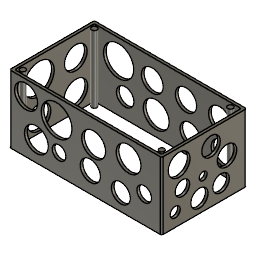
psu housing of anycibic kossel lienar plus_ (Autodesk Fusion 360 archive; units mm, degrees)
design "side_pannel"
part number: 2026-08-06-01-08-32-616
Autodesk Fusion 360 part; units mm, degrees
note: some values were not read from the file. Chosen so that the rebuilt part matches the saved one: which bodies a step acts on.
sketch "Sketch1" plane through (0, 0, 0) normal (0, 0, 1) x (1, 0, 0)
  line L0 (1, 0) -> (112, 0)
  line L1 (113, 0) -> (113, 63)
  line L2 (113, 63) -> (1, 63)
  line L3 (0, 63) -> (0, 1)
  line L4 (0, 0) -> (2, 0)
  line L5 (2, 3) -> (2, 60)
  line L6 (2, 63) -> (0, 63)
  line L7 (0, 62) -> (0, 0)
  line L8 (0, 0) -> (113, 0)
  line L9 (113, 0) -> (113, 2)
  line L10 (110, 2) -> (3, 2)
  line L11 (0, 2) -> (0, 0)
  line L12 (113, 63) -> (111, 63)
  line L13 (111, 60) -> (111, 3)
  line L14 (111, 0) -> (113, 0)
  line L15 (113, 1) -> (113, 62)
  line L16 (112, 63) -> (0, 63)
  line L17 (0, 63) -> (0, 61)
  line L18 (3, 61) -> (110, 61)
  line L19 (113, 61) -> (113, 63)
  arc A0 (112, 0) -> (113, 1) centre (112, 1) ccw
  arc A1 (113, 62) -> (112, 63) centre (112, 62) ccw
  arc A2 (1, 63) -> (0, 62) centre (1, 62) ccw
  arc A3 (0, 1) -> (1, 0) centre (1, 1) ccw
  arc A4 (3, 61) -> (2, 60) centre (3, 60) ccw
  arc A5 (2, 3) -> (3, 2) centre (3, 3) ccw
  arc A6 (110, 2) -> (111, 3) centre (110, 3) ccw
  arc A7 (111, 60) -> (110, 61) centre (110, 60) ccw
  dimension "d1" = 63
  dimension "d2" = 113
  dimension "d3" = 2
  dimension "d4" = 2
  dimension "d5" = 2
  dimension "d6" = 2
  dimension "d7" = 1
  dimension "d8" = 1
  constraint horizontal L0
  constraint vertical L1
  constraint horizontal L2
  constraint vertical L3
  constraint coincident L4.start L7.end
  constraint horizontal L4
  constraint vertical L5
  constraint horizontal L6
  constraint vertical L7
  constraint coincident L2 L6.start
  constraint horizontal L8
  constraint vertical L9
  constraint horizontal L10
  constraint vertical L11
  constraint coincident L1 L9.end
  constraint horizontal L12
  constraint vertical L13
  constraint horizontal L14
  constraint vertical L15
  constraint coincident L8 L14.start
  constraint horizontal L16
  constraint vertical L17
  constraint horizontal L18
  constraint vertical L19
  constraint coincident L7 L17.end
  constraint coincident L1.start L0
  constraint coincident L1.start L15
  constraint tangent L0 A0
  constraint tangent L15 A0
  constraint coincident L1.end L16
  constraint coincident L1.end L15
  constraint tangent L16 A1
  constraint tangent L15 A1
  constraint equal A0 A1
  constraint coincident L3.start L2
  constraint coincident L3.start L7
  constraint tangent L2 A2
  constraint tangent L7 A2
  constraint equal A0 A2
  constraint coincident L4.start L3
  constraint coincident L4.start L0
  constraint tangent L3 A3
  constraint tangent L0 A3
  constraint equal A0 A3
  constraint coincident L17.end L18
  constraint coincident L6.start L5
  constraint tangent L18 A4
  constraint tangent L5 A4
  constraint coincident L4.end L5
  constraint coincident L11.start L10
  constraint tangent L5 A5
  constraint tangent L10 A5
  constraint equal A4 A5
  constraint coincident L9.end L10
  constraint coincident L14.start L13
  constraint tangent L10 A6
  constraint tangent L13 A6
  constraint equal A4 A6
  constraint coincident L19.start L18
  constraint coincident L12.end L13
  constraint tangent L18 A7
  constraint tangent L13 A7
  constraint equal A4 A7
  measures "d1" distance of L4.start L3.start
  measures "d2" distance of L4.start L1.start
  measures "d3" distance of L3 L5
  measures "d4" distance of L0 L10
  measures "d5" distance of L13 L15
  measures "d6" distance of L2 L18
  measures "d7" radius of A0
  measures "d8" radius of A4
sketch "Sketch2" plane through (0, 0, 0) normal (0, 0, 1) x (1, 0, 0)
  circle A0 centre (108, 5) radius 2
  circle A1 centre (5, 5) radius 2
  circle A2 centre (106, 58) radius 2
  circle A3 centre (5, 58) radius 2
  line L0 (113, 1) -> (113, 62)
  line L1 (1, 0) -> (112, 0)
  line L2 (112, 63) -> (0, 63)
  line L3 (111, 60) -> (111, 3)
  line L4 (0, 62) -> (0, 0)
  dimension "d9" = 4
  dimension "d10" = 4
  dimension "d11" = 4
  dimension "d12" = 4
  dimension "d13" = 5
  dimension "d14" = 5
  dimension "d15" = 5
  dimension "d16" = 5
  dimension "d17" = 5
  dimension "d18" = 5
  dimension "d19" = 5
  dimension "d20" = 5
  measures "d9" diameter of A0
  measures "d10" diameter of A1
  measures "d11" diameter of A2
  measures "d12" diameter of A3
  measures "d13" distance of A0.centre L0
  measures "d14" distance of A0.centre L1
  measures "d15" distance of A2.centre L2
  measures "d16" distance of A2.centre L3
  measures "d17" distance of A3.centre L4
  measures "d18" distance of A3.centre L2
  measures "d19" distance of A1.centre L4
  measures "d20" distance of A1.centre L1
extrude "Extrude1" add sketch "Sketch2" sketch "Sketch1" along normal blind 50 of sketch 2 contours L0 L1 L2 L3 L4 L6 L7 L8 L9 L11 L12 L14 L15 L16 L17 L19 A0 A1 A2 A3 makes body 1 at (107.843, 58.7769, 33.3333) makes body 2 at (108.5417, 6.9252, 33.3333) makes body 3 at (6.9901, 57.8009, 16.6667) makes body 4 at (6.9901, 4.8009, 16.6667) makes body 5 at (75, 63, 16.6667)
sketch "Sketch3" plane through (0, 63, 0) normal (0, 1, 0) x (-1, 0, 0)
  line L0 (-112, 0) -> (-1, 0)
  line L1 (-1, 0) -> (-1, 50)
  line L2 (-1, 50) -> (-112, 50)
  line L3 (-112, 50) -> (-112, 0)
  circle A0 centre (-95, 35) radius 8.2335
  circle A1 centre (-70, 35) radius 7.862
  circle A2 centre (-45, 35) radius 8.0607
  circle A3 centre (-20, 35) radius 11.1803
  circle A4 centre (-96.9589, 14.4407) radius 8.2637
  circle A5 centre (-73.0876, 14.4407) radius 7.5151
  circle A6 centre (-47.8901, 14.4407) radius 9.578
  circle A7 centre (-24.9028, 14.4407) radius 6.4836
sketch "Sketch4" plane through (0, 0, 0) normal (-1, 0, 0) x (0, -1, 0)
  line L0 (-62, 0) -> (-1, 0)
  line L1 (-1, 0) -> (-1, 50)
  line L2 (-1, 50) -> (-62, 50)
  line L3 (-62, 50) -> (-62, 0)
  circle A0 centre (-47.1533, 34.4808) radius 8.5275
  circle A1 centre (-20.0401, 34.4808) radius 11.9074
  circle A2 centre (-47.1533, 12.6724) radius 9.578
  circle A3 centre (-20.0401, 10.3148) radius 8.6851
sketch "Sketch5" plane through (0, 0, 0) normal (0, -1, 0) x (1, 0, 0)
  line L0 (1, 0) -> (112, 0)
  line L1 (112, 0) -> (112, 50)
  line L2 (112, 50) -> (1, 50)
  line L3 (1, 50) -> (1, 0)
  circle A0 centre (12.3777, 38.9015) radius 8.5627
  circle A1 centre (35, 35) radius 11.3753
  circle A2 centre (62.4781, 33.0073) radius 8.8425
  circle A3 centre (88.4124, 36.8385) radius 9.1747
  circle A4 centre (100, 20) radius 5.3888
  circle A5 centre (82.6656, 12.083) radius 7.002
  circle A6 centre (60, 15) radius 7.449
  circle A7 centre (36.8385, 15) radius 5.0529
  circle A8 centre (20, 15) radius 8.8098
sketch "Sketch6" plane through (0, 0, 0) normal (-1, 0, 0) x (0, -1, 0)
  circle A0 centre (-20, 35) radius 11.232
  circle A1 centre (-47.3006, 35) radius 8.3691
  circle A2 centre (-21.8084, 9.7254) radius 5.5233
  circle A3 centre (-47.3006, 12.3777) radius 8.7945
extrude "Extrude2" cut sketch "Sketch3" against normal blind 2 contours A0 | A1 | A2 | A3 | A4 | A5 | A6 | A7 bodies 5
extrude "Extrude3" cut sketch "Sketch6" sketch "Sketch4" against normal blind 2 contours A0 | A1 | A3 of sketch 2 contours A3 bodies 5
extrude "Extrude4" cut sketch "Sketch5" against normal blind 2 contours A0 | A1 | A2 | A3 | A4 | A5 | A6 | A7 | A8 bodies 5
sketch "Sketch7" plane through (113, 0, 0) normal (1, 0, 0) x (0, 1, 0)
  line L0 (1, 0) -> (62, 0)
  line L1 (62, 0) -> (62, 50)
  line L2 (62, 50) -> (1, 50)
  line L3 (1, 50) -> (1, 0)
  circle A0 centre (12.9672, 38.9015) radius 8.0425
  circle A1 centre (36.6322, 38.9015) radius 6.8788
  circle A2 centre (48.4647, 27.0689) radius 7.2337
  circle A3 centre (28.0415, 9.8875) radius 6.3691
  circle A4 centre (15.3985, 22.6925) radius 5.3514
  circle A5 centre (30.797, 22.6925) radius 2.9176
  circle A6 centre (44.0883, 11.5083) radius 6.1166
  circle A7 centre (10.0495, 9.8875) radius 3.7281
extrude "Extrude5" cut sketch "Sketch7" against normal blind 2 contours A0 | A1 | A2 | A3 | A4 | A5 | A6 | A7 bodies 5

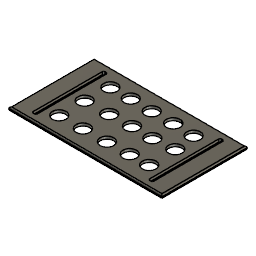
design "base"
part number: 2026-08-06-00-25-03-239
part number: 2026-08-06-00-26-41-990
Autodesk Fusion 360 part; units mm, degrees
sketch "Sketch1" plane through (0, 0, 0) normal (0, 0, 1) x (1, 0, 0) in component "base_layer"
  line L0 (0, 0) -> (113, 0)
  line L1 (113, 0) -> (113, 63)
  line L2 (113, 63) -> (0, 63)
  line L3 (0, 63) -> (0, 0)
  line L4 (9, 58) -> (12, 58)
  line L5 (104, 58) -> (101, 58)
  line L6 (13, 58) -> (14, 58)
  line L7 (15, 57) -> (15, 6)
  line L8 (14, 5) -> (13, 5)
  line L9 (12, 6) -> (12, 57)
  line L10 (100, 58) -> (99, 58)
  line L11 (98, 57) -> (98, 6)
  line L12 (99, 5) -> (100, 5)
  line L13 (101, 6) -> (101, 57)
  arc A0 (13, 58) -> (12, 57) centre (13, 57) ccw
  arc A1 (15, 57) -> (14, 58) centre (14, 57) ccw
  arc A2 (12, 6) -> (13, 5) centre (13, 6) ccw
  arc A3 (14, 5) -> (15, 6) centre (14, 6) ccw
  arc A4 (99, 58) -> (98, 57) centre (99, 57) ccw
  arc A5 (101, 57) -> (100, 58) centre (100, 57) ccw
  arc A6 (100, 5) -> (101, 6) centre (100, 6) ccw
  arc A7 (98, 6) -> (99, 5) centre (99, 6) ccw
  circle A8 centre (25, 50) radius 5
  circle A9 centre (25, 50) radius 5
  circle A10 centre (55.5469, 49.9659) radius 5
  circle A11 centre (71.1094, 50.2422) radius 5
  circle A12 centre (71.3194, 50.1842) radius 5
  circle A13 centre (86.6177, 49.7772) radius 5
  circle A14 centre (25, 50) radius 5
  circle A15 centre (24, 32) radius 5
  circle A16 centre (23.9972, 13.23) radius 5
  circle A17 centre (41.6022, 32.5064) radius 5
  circle A18 centre (41.1565, 13.5642) radius 5
  circle A19 centre (39.708, 50.3343) radius 5
  circle A20 centre (57.7588, 33.1749) radius 5
  circle A21 centre (73, 33) radius 5
  circle A22 centre (88.5119, 34.4006) radius 5
  circle A23 centre (58.4273, 14.0099) radius 5
  circle A24 centre (74.8067, 14.4556) radius 5
  circle A25 centre (88.9576, 14.6785) radius 5
  point P0 (15, 58)
  point P1 (15, 5)
  point P2 (98, 58)
  dimension "d1" = 113
  dimension "d2" = 63
  dimension "d5" = 5
  dimension "d7" = 5
  dimension "d14" = 3
  dimension "d15" = 5
  dimension "d16" = 3
  dimension "d17" = 5
  dimension "d18" = 1
  dimension "d19" = 1
  dimension "d20" = 1
  dimension "d21" = 1
  dimension "d22" = 10
  dimension "d23" = 10
  dimension "d24" = 10
  dimension "d25" = 10
  dimension "d26" = 10
  dimension "d27" = 10
  dimension "d28" = 10
  dimension "d29" = 10
  dimension "d30" = 10
  dimension "d31" = 10
  dimension "d32" = 10
  dimension "d33" = 10
  dimension "d34" = 10
  dimension "d35" = 10
  dimension "d36" = 10
  dimension "d37" = 10
  dimension "d38" = 10
  dimension "d39" = 10
  constraint horizontal L0
  constraint vertical L1
  constraint horizontal L2
  constraint vertical L3
  constraint coincident L0.start L3.end
  constraint horizontal L6
  constraint vertical L7
  constraint horizontal L8
  constraint vertical L9
  constraint horizontal L10
  constraint vertical L11
  constraint horizontal L12
  constraint vertical L13
  constraint coincident L4.end L9
  constraint coincident L4.end L6
  constraint tangent L9 A0
  constraint tangent L6 A0
  constraint coincident P0 L6
  constraint coincident P0 L7
  constraint tangent L6 A1
  constraint tangent L7 A1
  constraint tangent L8 A2
  constraint tangent L9 A2
  constraint equal A1 A2
  constraint coincident P1 L8
  constraint coincident P1 L7
  constraint tangent L8 A3
  constraint tangent L7 A3
  constraint coincident P2 L10
  constraint coincident P2 L11
  constraint tangent L10 A4
  constraint tangent L11 A4
  constraint coincident L5.end L13
  constraint coincident L5.end L10
  constraint tangent L13 A5
  constraint tangent L10 A5
  constraint equal A4 A5
  constraint tangent L13 A6
  constraint tangent L12 A6
  constraint equal A4 A6
  constraint tangent L11 A7
  constraint tangent L12 A7
  constraint equal A4 A7
  measures "d1" distance of L0.start L0.end
  measures "d2" distance of L0.start L2.end
  measures "d5" distance of L2 L4.start
  measures "d7" distance of L2 L5.start
  measures "d14" distance of L4.end P0
  measures "d15" distance of L0 P1
  measures "d16" distance of L5.end P2
  measures "d17" distance of L0 L12
  measures "d18" radius of A0
  measures "d19" radius of A1
  measures "d20" radius of A3
  measures "d21" radius of A4
  measures "d22" diameter of A8
  measures "d23" diameter of A9
  measures "d24" diameter of A10
  measures "d25" diameter of A11
  measures "d26" diameter of A12
  measures "d27" diameter of A13
  measures "d28" diameter of A14
  measures "d29" diameter of A15
  measures "d30" diameter of A16
  measures "d31" diameter of A17
  measures "d32" diameter of A18
  measures "d33" diameter of A19
  measures "d34" diameter of A20
  measures "d35" diameter of A21
  measures "d36" diameter of A22
  measures "d37" diameter of A23
  measures "d38" diameter of A24
  measures "d39" diameter of A25
extrude "Extrude1" add sketch "Sketch1" along normal blind 2 in component "base_layer"
fillet "Fillet1" radius 1 4 edges at (113, 31.5, 2) (56.5, 63, 2) (0, 31.5, 2) (56.5, 0, 2) in component "base_layer"
component "base_layer" placed x (1, 0, 0) y (0, 1, 0) z (0, 0, 1) at (0, 0, 0)
